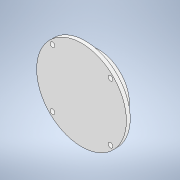
# Autodesk Inventor part: Chapeau Haut.stl
Saved by Autodesk Inventor 2022 (Build 260153000, 153)
## iProperties
Created: 2021-12-06
Part Number: Chapeau Haut.stl
Material: Générique
Document SubType Name: Modeling
Designer: utilisateur
Density: 1 g/cm^3
Appearance: Par défaut(1)
Author: utilisateur
Autodesk Inventor part; units mm, degrees
ref_plane "YZ Plane" through (0, 0, 0) normal (1, 0, 0) x (0, 1, 0)
ref_plane "XZ Plane" through (0, 0, 0) normal (0, 1, 0) x (-1, 0, 0)
ref_plane "XY Plane" through (0, 0, 0) normal (0, 0, 1) x (1, 0, 0)
sketch "Esquisse1" plane through (0, 0, 0) normal (0, 0, 1) x (1, 0, 0)
  circle A0 centre (0, 0) radius 58.033
  circle A1 centre (0, 0) radius 53.033 construction
  line L0 (37.5, -37.5) -> (-37.5, -37.5) construction
  line L1 (-37.5, -37.5) -> (-37.5, 37.5) construction
  line L2 (-37.5, 37.5) -> (37.5, 37.5) construction
  line L3 (37.5, 37.5) -> (37.5, -37.5) construction
  line L4 (37.5, -37.5) -> (-37.5, 37.5) construction
  line L5 (-37.5, -37.5) -> (37.5, 37.5) construction
  circle A2 centre (-37.5, 37.5) radius 3.1
  circle A3 centre (37.5, 37.5) radius 3.1
  circle A4 centre (37.5, -37.5) radius 3.1
  circle A5 centre (-37.5, -37.5) radius 3.1
  dimension "d0" = 116.066
  dimension "d2" = 106.066
  dimension "d22" = 6.2
  dimension "d23" = 75
  dimension "d24" = 5
  constraints: 12 end point, 6 centre point, 5 coincident, 3 equal radius, 2 midpoint, 2 parallel, 2 perpendicular, 2 point on circle, 1 horizontal, 1 point on line
  measures "d0" diameter of A0
  measures "d2" diameter of A1
  measures "d22" diameter of A2
  measures "d23" distance of L1.end L2.end
  measures "d24" radial gap between concentric circles of A0 A1
extrude "Extrusion1" add sketch "Esquisse1" along normal mid plane 5
sketch "Esquisse2" plane through (0, 0, -2.5) normal (0, 0, -1) x (-1, 0, 0)
  circle A0 centre (0, 0) radius 40
  dimension "d6" = 80
  constraints: 1 centre point, 1 coincident
  measures "d6" diameter of A0
extrude "Extrusion2" add sketch "Esquisse2" along normal blind 17
